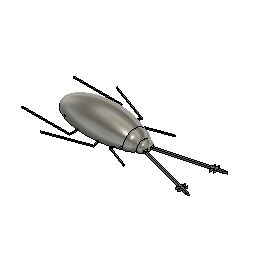
Roach_v1 (Autodesk Fusion 360 design; units mm, degrees)
part number: 2026-05-05-08-31-05-586
Autodesk Fusion 360 part; units mm, degrees
sketch "Sketch1" plane through (0, 0, 0) normal (0, 1, 0) x (1, 0, 0)
  spline S0 degree 5 poles (0, 0) (0, -0.8883) (0.3538, -2.6533) (1.9458, -5.2658) (6.0893, -8.6064) (14.0532, -12.1437) (24.0002, -14.56) (35, -15.4332) (45.9998, -14.56) (55.9468, -12.1437) (63.9107, -8.6064) (68.0542, -5.2658) (69.6462, -2.6533) (70, -0.8883) (70, 0) knots 0 0 0 0 0 0 0.1 0.2 0.3 0.4 0.5 0.6 0.7 0.8 0.9 1 1 1 1 1 1
  line L0 (70, 0) -> (0, 0)
  line L1 (70, -3.25) -> (70, 3.25)
  line L2 (0, 3.25) -> (0, -3.25)
  line L3 (35, 0) -> (35, -21) construction
  line L4 (25, -15) -> (45, -15)
  point P0 (35, -15)
  dimension "d1" = 70
  dimension "d2" = 15
  dimension "d3" = 20
  dimension "d4" = 6.5
  dimension "d5" = 6.5
  constraint horizontal L0
  constraint midpoint S0.end L1
  constraint perpendicular L0 L1
  constraint midpoint S0.start L2
  constraint perpendicular L0 L2
  constraint midpoint L0 L3.start
  constraint perpendicular L0 L3
  constraint coincident S0.start L0.end
  constraint coincident P0 L3
  constraint midpoint P0 L4
  constraint perpendicular L3 L4
  measures "d1" distance of S0.start S0.end
  measures "d2" distance of P0 L0
  measures "d3" distance of L4.start L4.end
  measures "d4" distance of L1.start L1.end
  measures "d5" distance of L2.start L2.end
revolve "Revolve1" add sketch "Sketch1" angle 180 about axis through (70, 0, 0) along (-1, 0, 0)
sketch "Sketch2" plane through (0, 0, 0) normal (0, 1, 0) x (1, 0, 0)
  line L0 (0, 0) -> (70, 0) construction
  spline S0 degree 5 poles (65, 0) (65, 0.6131) (65.0493, 1.744) (65.2712, 3.1542) (65.8047, 4.4857) (66.5579, 5.3974) (67.0619, 5.827) (67.0623, 6.1354) (66.5723, 6.8361) (65.5527, 7.9373) (64.0281, 9.1779) (62.0963, 10.1549) (60.1158, 10.4434) (58.4644, 9.8281) (57.2442, 8.328) (56.4671, 6.0781) (56.1409, 3.8325) (56.0256, 1.9744) (56, 0.6692) (56, 0) knots 0 0 0 0 0 0 0.066667 0.133333 0.2 0.266667 0.333333 0.4 0.466667 0.533333 0.6 0.666667 0.733333 0.8 0.866667 0.933333 1 1 1 1 1 1
  line L1 (56, 0) -> (65, 0)
  line L2 (56, 3) -> (56, -3)
  line L3 (65, -4) -> (65, 4)
  line L4 (67, 5.5) -> (67, 6.5)
  line L5 (63.7078, 9.4883) -> (60.3608, 10.5117)
  spline S1 degree 5 poles (65, 0) (65, 0.4374) (65.0263, 1.2851) (65.1447, 2.475) (65.469, 3.8801) (66.1892, 5.2313) (67.2183, 6.0751) (68.5, 6.3309) (69.7817, 6.0622) (70.8108, 5.3603) (71.531, 4.1885) (71.8553, 2.8245) (71.9737, 1.5248) (72, 0.5297) (72, 0) knots 0 0 0 0 0 0 0.1 0.2 0.3 0.4 0.5 0.6 0.7 0.8 0.9 1 1 1 1 1 1
  line L6 (65, 0) -> (72, 0)
  line L7 (68.5, 6.2) -> (68.5, 0) construction
  spline S2 degree 5 poles (0, 0) (0, 0.8883) (0.3538, 2.6533) (1.9458, 5.2658) (6.0893, 8.6064) (14.0532, 12.1437) (24.0002, 14.56) (35, 15.4332) (45.9998, 14.56) (55.9468, 12.1437) (63.9107, 8.6064) (68.0542, 5.2658) (69.6462, 2.6533) (70, 0.8883) (70, 0) knots 0 0 0 0 0 0 0.1 0.2 0.3 0.4 0.5 0.6 0.7 0.8 0.9 1 1 1 1 1 1
  line L8 (72, 1.7874) -> (72, -1.7874)
  line L9 (65, -1.476) -> (65, 1.476)
  line L10 (67.7779, 6.2) -> (69.2221, 6.2)
  point P0 (67, 6)
  point P1 (62.0343, 10)
  point P2 (68.5, 6.2)
  dimension "d7" = 9
  dimension "d9" = 6
  dimension "d10" = 8
  dimension "d11" = 1
  dimension "d12" = 6
  dimension "d13" = 3.5
  dimension "d14" = 17
  dimension "d15" = 10
  dimension "d16" = 7
  dimension "d17" = 5
  dimension "d18" = 6.2
  constraint coincident L0.start S2.start
  constraint horizontal L0
  constraint coincident L0 S0.start
  constraint coincident L0 S0.end
  constraint midpoint S0.end L2
  constraint perpendicular L0 L2
  constraint midpoint S0.start L3
  constraint perpendicular L1 L3
  constraint midpoint P0 L4
  constraint perpendicular L0 L4
  constraint midpoint P1 L5
  constraint perpendicular L3 L6
  constraint coincident P2 L7.start
  constraint coincident L6 L7.end
  constraint perpendicular L6 L7
  constraint midpoint L6 L7.end
  constraint coincident L0.end S2
  constraint midpoint S1.end L8
  constraint perpendicular L6 L8
  constraint midpoint S0.start L9
  constraint perpendicular L6 L9
  constraint midpoint P2 L10
  constraint perpendicular L7 L10
  measures "d7" distance of S0.start S0.end
  measures "d9" distance of L2.start L2.end
  measures "d10" distance of L3.start L3.end
  measures "d11" distance of L4.start L4.end
  measures "d12" vertical distance of L0.end P0
  measures "d13" distance of L5.start L5.end
  measures "d14" angle of L0 L5
  measures "d15" distance of P1 L1
  measures "d16" distance of S0.start S1.end
  measures "d17" distance of L0.end L3
  measures "d18" distance of P2 L7.end
revolve "Revolve2" add sketch "Sketch2" angle 180 about axis through (0, 0, 0) along (1, 0, 0) contours S0 L1 S1 S2 | S0 S1 L6 S2 | L4 S1 L6 S2 | S0 S2 | L4 S1 S2
sketch "Sketch3" plane through (0, 0, 0) normal (0, 0, 1) x (1, 0, 0)
  line L0 (0, 0) -> (72, 0) construction
  line L1 (72, 0) -> (71, 0)
  line L2 (36, 0) -> (36, 1) construction
  spline S0 degree 5 poles (36, 1) (36.2369, 1) (36.7103, 0.9872) (37.4188, 0.9297) (38.3523, 0.7878) (39.4471, 0.5447) (40.1995, 0.3275) (40.6512, 0.1631) (40.8935, 0.0543) (41, 0) knots 0 0 0 0 0 0 0.2 0.4 0.6 0.8 1 1 1 1 1 1
  line L3 (40.7772, 0.1135) -> (41.2228, -0.1135)
  line L4 (35.5, 1) -> (36.5, 1)
  line L5 (36, 1) -> (36, 4) construction
  spline S1 degree 5 poles (36, 4) (36.7891, 4) (38.3542, 3.9458) (40.6629, 3.7019) (43.6392, 3.1027) (47.0006, 2.0937) (49.1519, 1.2233) (50.2913, 0.5951) (50.8048, 0.1952) (51, 0) knots 0 0 0 0 0 0 0.2 0.4 0.6 0.8 1 1 1 1 1 1
  line L6 (50.6464, 0.3536) -> (51.3536, -0.3536)
  line L7 (34.5, 4) -> (37.5, 4)
  line L8 (41, 0) -> (51, 0)
  line L9 (36, 1) -> (36, 4) construction
  spline S2 degree 5 poles (36, 4) (35.2109, 4) (33.6458, 3.9458) (31.3371, 3.7019) (28.3608, 3.1027) (24.9994, 2.0937) (22.8481, 1.2233) (21.7087, 0.5951) (21.1952, 0.1952) (21, 0) knots 0 0 0 0 0 0 0.2 0.4 0.6 0.8 1 1 1 1 1 1
  line L10 (37.5, 4) -> (34.5, 4)
  line L11 (21.3536, 0.3536) -> (20.6464, -0.3536)
  spline S3 degree 5 poles (36, 1) (35.7631, 1) (35.2897, 0.9872) (34.5812, 0.9297) (33.6477, 0.7878) (32.5529, 0.5447) (31.8005, 0.3275) (31.3488, 0.1631) (31.1065, 0.0543) (31, 0) knots 0 0 0 0 0 0 0.2 0.4 0.6 0.8 1 1 1 1 1 1
  line L12 (36.5, 1) -> (35.5, 1)
  line L13 (31.2228, 0.1135) -> (30.7772, -0.1135)
  line L14 (31, 0) -> (21, 0)
  dimension "d20" = 72
  dimension "d21" = 1
  dimension "d22" = 5
  dimension "d23" = 27
  dimension "d24" = 45
  dimension "d25" = 1
  dimension "d26" = 3
  dimension "d27" = 0.5
  dimension "d28" = 1
  dimension "d29" = 10
  dimension "d30" = 3
  constraint coincident L0.start origin
  constraint horizontal L0
  constraint coincident L0 L1.end
  constraint midpoint L0 L2.start
  constraint perpendicular L0 L2
  constraint coincident L0 S0.end
  constraint midpoint S0.end L3
  constraint midpoint L2.end L4
  constraint parallel L2 L5
  constraint midpoint S1.end L6
  constraint midpoint L5.end L7
  constraint parallel L0 L8
  constraint symmetric L2.end L5 S0.start
  constraint symmetric S0.end L5 S3.end
  constraint symmetric L3.start L5 L13.start
  constraint symmetric L3.end L5 L13.end
  constraint symmetric L4.start L5 L4.end
  constraint symmetric L4.end L5 L4.start
  constraint symmetric S1.start L5 L9.end
  constraint symmetric L5 S1.end S2.end
  constraint symmetric L5 L6.start L11.start
  constraint symmetric L5 L6.end L11.end
  constraint symmetric L5 L7.start L7.end
  constraint symmetric L5 L7.end L7.start
  measures "d20" distance of L0.start L0.end
  measures "d21" distance of L2.start L2.end
  measures "d22" distance of L2 S0.end
  measures "d23" angle of L0 L3
  measures "d24" angle of L0 L6
  measures "d25" distance of L4.start L4.end
  measures "d26" distance of L7.start L7.end
  measures "d27" distance of L3.start L3.end
  measures "d28" distance of L6.start L6.end
  measures "d29" distance of S0.end S1.end
  measures "d30" distance of L2.end L5.end
sketch "Sketch4" plane through (0, 0, 0) normal (0, 0, 1) x (1, 0, 0)
  line L0 (0, 0) -> (13, 0) construction
  line L1 (13, 0) -> (13, 1.5) construction
  circle A0 centre (13, 1.5) radius 0.7
  line L2 (36, 1) -> (36, 4)
  line L3 (59, 0) -> (59, 1.5) construction
  line L4 (72, 0) -> (59, 0) construction
  circle A1 centre (59, 1.5) radius 0.7
  point P0 (72, 0)
  dimension "d31" = 13
  dimension "d32" = 1.5
  dimension "d33" = 1.4
  constraint coincident L0.start origin
  constraint horizontal L0
  constraint perpendicular L0 L1
  constraint coincident L1.end A0.centre
  constraint symmetric L0.start L2 L4.start
  constraint symmetric L0.start L2 P0
  constraint symmetric L0.end L2 L3.start
  constraint symmetric L1.end L2 L3.end
  constraint symmetric A0 L2 A1
  measures "d31" distance of L0.start L0.end
  measures "d32" distance of L0.end L1.end
  measures "d33" diameter of A0
extrude "Extrude1" cut sketch "Sketch4" along normal mid plane 40
sketch "Sketch5" plane through (0, 0, 0) normal (0, 1, 0) x (1, 0, 0)
  line L0 (72, 0) -> (70, 0) construction
  line L1 (70, 0) -> (70, 1.5) construction
  line L2 (70, 1.5) -> (118.2963, 14.441)
  line L3 (118.2963, 14.441) -> (117.9081, 15.8898)
  line L4 (117.9081, 15.8898) -> (69.6118, 2.9489)
  line L5 (69.6118, 2.9489) -> (70, 1.5)
  line L6 (118.2963, 14.441) -> (120.8058, 15.8898)
  line L7 (120.8058, 15.8898) -> (117.9081, 15.8898)
  line L8 (114.4326, 13.4057) -> (114.4326, 10.5079)
  line L9 (114.4326, 10.5079) -> (112.9837, 13.0174)
  line L10 (112.0178, 9.8609) -> (110.5689, 12.3704)
  line L11 (112.0178, 12.7586) -> (112.0178, 9.8609)
  line L12 (118.1022, 15.1654) -> (69.8059, 2.2244) construction
  line L13 (114.0444, 14.8546) -> (112.5955, 17.3641)
  line L14 (112.5955, 17.3641) -> (112.5955, 14.4663)
  line L15 (111.6295, 14.2075) -> (110.1807, 16.7171)
  line L16 (110.1807, 16.7171) -> (110.1807, 13.8193)
  line L17 (72, 0) -> (71, 0)
  line L18 (114.4326, -10.5079) -> (112.9837, -13.0174)
  line L19 (120.8058, -15.8898) -> (117.9081, -15.8898)
  line L20 (70, -1.5) -> (118.2963, -14.441)
  line L21 (112.0178, -9.8609) -> (110.5689, -12.3704)
  line L22 (118.2963, -14.441) -> (120.8058, -15.8898)
  line L23 (112.5955, -17.3641) -> (112.5955, -14.4663)
  line L24 (112.0178, -12.7586) -> (112.0178, -9.8609)
  line L25 (118.2963, -14.441) -> (117.9081, -15.8898)
  line L26 (114.4326, -13.4057) -> (114.4326, -10.5079)
  line L27 (118.1022, -15.1654) -> (69.8059, -2.2244) construction
  line L28 (114.0444, -14.8546) -> (112.5955, -17.3641)
  line L29 (110.1807, -16.7171) -> (110.1807, -13.8193)
  line L30 (111.6295, -14.2075) -> (110.1807, -16.7171)
  line L31 (117.9081, -15.8898) -> (69.6118, -2.9489)
  line L32 (69.6118, -2.9489) -> (70, -1.5)
  point P0 (72, 0)
  dimension "d36" = 1.5
  dimension "d37" = 2
  dimension "d39" = 50
  dimension "d40" = 50
  dimension "d41" = 105
  dimension "d42" = 1.5
  dimension "d43" = 75
  dimension "d44" = 75
  dimension "d45" = 75
  dimension "d46" = 75
  dimension "d47" = 1.5
  dimension "d48" = 4
  dimension "d49" = 1.5
  dimension "d50" = 1
  dimension "d51" = 75
  constraint horizontal L0
  constraint perpendicular L0 L1
  constraint coincident P0 L0.start
  constraint perpendicular L2 L3
  constraint perpendicular L3 L4
  constraint coincident L2 L8.start
  constraint coincident L2 L9.end
  constraint coincident L2 L11.start
  constraint vertical L11
  constraint coincident L2 L10.end
  constraint midpoint L3 L12.start
  constraint perpendicular L3 L12
  constraint midpoint L5 L12.end
  constraint symmetric L8.start L12 L13.start
  constraint symmetric L8.end L12 L13.end
  constraint symmetric L9.end L12 L14.end
  constraint symmetric L10.end L12 L16.end
  constraint symmetric L10.start L12 L15.end
  constraint symmetric L11.start L12 L15.start
  constraint symmetric L1.end L17 L20.start
  constraint symmetric L2.end L17 L20.end
  constraint symmetric L3.end L17 L19.end
  constraint symmetric L4.end L17 L31.end
  constraint symmetric L6.end L17 L19.start
  constraint symmetric L8.start L17 L26.start
  constraint symmetric L8.end L17 L18.start
  constraint symmetric L9.end L17 L18.end
  constraint symmetric L10.end L17 L21.end
  constraint symmetric L10.start L17 L21.start
  constraint symmetric L11.start L17 L24.start
  constraint symmetric L12.start L17 L27.start
  constraint symmetric L12.end L17 L27.end
  constraint symmetric L14.end L17 L23.end
  constraint symmetric L13.start L17 L28.start
  constraint symmetric L15.end L17 L29.start
  constraint symmetric L13.end L17 L23.start
  constraint symmetric L15.start L17 L30.start
  constraint symmetric L16.end L17 L29.end
  measures "d36" distance of L0.end L1.end
  measures "d37" distance of P0 L0.end
  measures "d39" distance of L1.end L2.end
  measures "d40" distance of L3.end L4.end
  measures "d41" angle of L1 L2
  measures "d42" distance of L2.end L3.end
  measures "d43" angle of L3 L6
  measures "d44" angle of L3 L7
  measures "d45" angle of L2 L8
  measures "d46" angle of L2 L9
  measures "d47" distance of L8.start L9.end
  measures "d48" distance of L2.end L8.start
  measures "d49" distance of L10.end L11.start
  measures "d50" distance of L9.end L11.start
  measures "d51" angle of L2 L10
extrude "Extrude2" add sketch "Sketch5" along normal blind 1.5
fillet "Fillet1" radius 0.8 6 edges at (71.6172, 0.7516, 3.4862) (71.727, 1.5, 2.7506) (71.8905, 0.7499, -2.0065) (71.7296, 1.5, -2.737) (71.8904, 0.7516, 2.0065) (71.6171, 0.752, -3.4862)
extrude "Extrude3" cut sketch "Sketch3" along normal mid plane 10
sketch "Sketch6" plane through (0, 0, 0) normal (0, 1, 0) x (1, 0, 0)
  line L0 (0, 0) -> (72, 0) construction
  line L1 (27, 0) -> (27, 12) construction
  line L2 (27, 12) -> (27, 21)
  line L3 (27, 21) -> (-12.2, 21)
  line L4 (-12.2, 21) -> (-12.2, 21.8)
  line L5 (-12.2, 21.8) -> (27.8, 21.8)
  line L6 (27.8, 21.8) -> (27.8, 12)
  line L7 (27, 12) -> (27.8, 12)
  line L8 (13.2567, 31.2749) -> (13.5303, 32.0267)
  line L9 (45.3941, 19.5778) -> (13.2567, 31.2749)
  line L10 (46.4195, 20.056) -> (43.7518, 12.7264)
  line L11 (43, 13) -> (45.3941, 19.5778)
  line L12 (13.5303, 32.0267) -> (46.4195, 20.056)
  line L13 (43, 13) -> (43.7518, 12.7264)
  line L14 (43, 0) -> (43, 13) construction
  line L15 (54.3153, 14.2203) -> (55.7518, 10.2736)
  line L16 (55, 10) -> (53.2899, 14.6985)
  line L17 (53.2899, 14.6985) -> (72.0838, 21.5389)
  line L18 (55, 0) -> (55, 10) construction
  line L19 (55, 10) -> (55.7518, 10.2736)
  line L20 (72.3574, 20.7871) -> (54.3153, 14.2203)
  line L21 (72.0838, 21.5389) -> (72.3574, 20.7871)
  line L22 (27, -12) -> (27, -21)
  line L23 (46.4195, -20.056) -> (43.7518, -12.7264)
  line L24 (27, -12) -> (27.8, -12)
  line L25 (27, -21) -> (-12.2, -21)
  line L26 (72.0838, -21.5389) -> (72.3574, -20.7871)
  line L27 (55, -10) -> (53.2899, -14.6985)
  line L28 (55, -10) -> (55.7518, -10.2736)
  line L29 (-12.2, -21.8) -> (27.8, -21.8)
  line L30 (13.2567, -31.2749) -> (13.5303, -32.0267)
  line L31 (72.3574, -20.7871) -> (54.3153, -14.2203)
  line L32 (54.3153, -14.2203) -> (55.7518, -10.2736)
  line L33 (45.3941, -19.5778) -> (13.2567, -31.2749)
  line L34 (13.5303, -32.0267) -> (46.4195, -20.056)
  line L35 (-12.2, -21) -> (-12.2, -21.8)
  line L36 (53.2899, -14.6985) -> (72.0838, -21.5389)
  line L37 (43, -13) -> (43.7518, -12.7264)
  line L38 (43, -13) -> (45.3941, -19.5778)
  line L39 (27.8, -21.8) -> (27.8, -12)
  line L40 (0, 0) -> (72, 0) construction
  dimension "d58" = 72
  dimension "d59" = 27
  dimension "d60" = 12
  dimension "d61" = 9
  dimension "d63" = 0.8
  dimension "d64" = 0.8
  dimension "d65" = 40
  dimension "d70" = 7
  dimension "d71" = 0.8
  dimension "d72" = 0.8
  dimension "d73" = 35
  dimension "d74" = 13
  dimension "d75" = 16
  dimension "d76" = 160
  dimension "d77" = 5
  dimension "d78" = 0.8
  dimension "d81" = 10
  dimension "d82" = 200
  dimension "d83" = 0.8
  dimension "d85" = 20
  dimension "d86" = 12
  constraint coincident L0.start L40.start
  constraint horizontal L0
  constraint coincident L0 L1.start
  constraint perpendicular L0 L1
  constraint perpendicular L2 L3
  constraint perpendicular L3 L4
  constraint perpendicular L3 L6
  constraint perpendicular L2 L7
  constraint perpendicular L5 L6
  constraint parallel L1 L2
  constraint perpendicular L9 L11
  constraint perpendicular L8 L9
  constraint perpendicular L9 L10
  constraint perpendicular L11 L13
  constraint perpendicular L10 L12
  constraint coincident L0 L14.start
  constraint perpendicular L0 L14
  constraint perpendicular L16 L17
  constraint perpendicular L17 L21
  constraint perpendicular L15 L17
  constraint perpendicular L16 L19
  constraint perpendicular L15 L20
  constraint coincident L0 L18.start
  constraint perpendicular L0 L18
  constraint symmetric L40.start L0 origin
  constraint symmetric L40.end L0 L0.end
  constraint symmetric L0 L1.end L22.start
  constraint symmetric L0 L2.end L22.end
  constraint symmetric L0 L3.end L25.end
  constraint symmetric L0 L4.end L29.start
  constraint symmetric L0 L5.end L29.end
  constraint symmetric L0 L6.end L24.end
  constraint symmetric L0 L8.start L30.start
  constraint symmetric L0 L9.start L33.start
  constraint symmetric L0 L11.start L37.start
  constraint symmetric L0 L8.end L30.end
  constraint symmetric L0 L10.end L23.end
  constraint symmetric L0 L10.start L23.start
  constraint symmetric L0 L15.end L28.end
  constraint symmetric L0 L15.start L31.end
  constraint symmetric L0 L20.start L26.end
  constraint symmetric L0 L16.end L27.end
  constraint symmetric L0 L17.end L26.start
  constraint symmetric L0 L16.start L27.start
  measures "d58" distance of L0.start L0.end
  measures "d59" distance of L0.start L1.start
  measures "d60" distance of L1.start L1.end
  measures "d61" distance of L1.end L2.end
  measures "d63" distance of L2 L6
  measures "d64" distance of L3 L5
  measures "d65" distance of L4.end L5.end
  measures "d70" distance of L9.start L11.start
  measures "d71" distance of L10 L11
  measures "d72" distance of L9 L12
  measures "d73" distance of L8.end L10.start
  measures "d74" distance of L11.start L14.start
  measures "d75" distance of L1.start L14.start
  measures "d76" angle of L11 L14
  measures "d77" distance of L16.end L16.start
  measures "d78" distance of L15 L16
  measures "d81" distance of L18.start L16.start
  measures "d83" distance of L17 L20
  measures "d85" distance of L16.end L17.end
  measures "d86" distance of L14.start L18.start
extrude "Extrude4" add sketch "Sketch6" along normal blind 0.8
